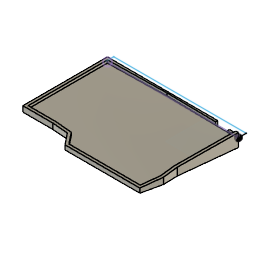
newcase v2 (Autodesk Fusion 360 design; units mm, degrees)
Autodesk Fusion 360 part; units mm, degrees
sketch "board" plane through (0, 0, 0) normal (0, 0, 1) x (1, 0, 0)
  line L0 (-11.43, -11.43) -> (-11.43, 76.4948)
  line L1 (-11.43, 76.4948) -> (53.2209, 77.7986)
  line L2 (53.2209, 77.7986) -> (127.9595, 76.6452)
  line L3 (127.9595, 76.6452) -> (127.335, 12)
  line L4 (127.335, 12) -> (129.2793, -5.0449)
  line L5 (129.2793, -5.0449) -> (126.9476, -25.6233)
  line L6 (126.9476, -25.6233) -> (47.9467, -25.6233)
  line L7 (47.9467, -25.6233) -> (38, -13.05)
  line L8 (38, -13.05) -> (19, -11.43)
  line L9 (19, -11.43) -> (-11.43, -11.43)
  line L10 (130.3366, 12.1561) -> (132.2986, -5.0438)
  line L11 (132.2986, -5.0438) -> (129.6269, -28.6233)
  line L12 (129.6269, -28.6233) -> (46.4947, -28.6233)
  line L13 (46.4947, -28.6233) -> (36.4523, -15.9289)
  line L14 (36.4523, -15.9289) -> (18.8723, -14.43)
  line L15 (18.8723, -14.43) -> (-14.43, -14.43)
  line L16 (-14.43, -14.43) -> (-14.43, 79.4349)
  line L17 (-14.43, 79.4349) -> (53.2138, 80.799)
  line L18 (53.2138, 80.799) -> (130.9882, 79.5988)
  line L19 (130.9882, 79.5988) -> (130.3366, 12.1561)
  line L20 (-35, 100) -> (162.96, 100)
  line L21 (162.96, 100) -> (162.96, -48.8802)
  line L22 (162.96, -48.8802) -> (-35, -48.8802)
  line L23 (-35, -48.8802) -> (-35, 100)
  dimension "d1" = -3
  constraint horizontal L6
  constraint vertical L0
  constraint horizontal L20
  constraint vertical L21
  constraint horizontal L22
  constraint vertical L23
sketch "cutout" plane through (0, 0, 0) normal (0, 0, 1) x (1, 0, 0)
  line L0 (-7.525, -11.025) -> (26.525, -11.025)
  line L1 (-10.525, -8.025) -> (-10.525, 65.025)
  line L2 (-7.525, 68.025) -> (27.475, 68.025)
  line L3 (29.525, -8.025) -> (29.525, -5.025)
  line L4 (29.525, -5.025) -> (43.375, -5.025)
  line L5 (46.475, 74.025) -> (30.475, 74.025)
  line L6 (27.475, 71.025) -> (27.475, 68.025)
  line L7 (67.525, 74.025) -> (67.525, 77.025)
  line L8 (67.525, 77.025) -> (46.475, 77.025)
  line L9 (46.475, 77.025) -> (46.475, 74.025)
  line L10 (86.425, -5.025) -> (87.0325, -5.025)
  line L11 (67.525, 74.025) -> (102.525, 74.025)
  line L12 (105.525, -2.6875) -> (105.525, 0.975)
  line L13 (105.525, 26.025) -> (105.525, 71.025)
  line L14 (105.525, 0.975) -> (107.9545, 0.975)
  line L15 (110.9113, 0.975) -> (121.525, 0.975)
  line L16 (124.525, 3.975) -> (124.525, 20.025)
  line L17 (121.525, 23.025) -> (108.525, 23.025)
  line L18 (49.375, -24.025) -> (86.425, -24.025)
  line L19 (46.375, -8.025) -> (46.375, -21.025)
  line L20 (86.425, -24.025) -> (86.425, -23.1507)
  line L21 (86.425, -11.969) -> (86.425, -5.025)
  line L22 (86.425, -23.1507) -> (103.4355, -24.6389)
  line L23 (106.6855, -21.9118) -> (106.7904, -20.7125)
  line L24 (107.4166, -2.853) -> (105.525, -2.6875)
  line L25 (87.0325, -5.025) -> (86.425, -11.969)
  line L26 (106.7904, -20.7125) -> (122.8174, -22.965)
  line L27 (126.2057, -20.4117) -> (128.4394, -4.5179)
  line L28 (125.8862, -1.1296) -> (110.9113, 0.975)
  line L29 (107.9545, 0.975) -> (107.4166, -2.853)
  arc A0 (26.525, -11.025) -> (29.525, -8.025) centre (26.525, -8.025) ccw
  arc A1 (46.375, -8.025) -> (43.375, -5.025) centre (43.375, -8.025) ccw
  arc A2 (46.375, -21.025) -> (49.375, -24.025) centre (49.375, -21.025) ccw
  arc A3 (103.4355, -24.6389) -> (106.6855, -21.9118) centre (103.6969, -21.6503) ccw
  arc A4 (122.8174, -22.965) -> (126.2057, -20.4117) centre (123.2349, -19.9942) ccw
  arc A5 (128.4394, -4.5179) -> (125.8862, -1.1296) centre (125.4686, -4.1004) ccw
  arc A6 (121.525, 0.975) -> (124.525, 3.975) centre (121.525, 3.975) ccw
  arc A7 (124.525, 20.025) -> (121.525, 23.025) centre (121.525, 20.025) ccw
  arc A8 (105.525, 26.025) -> (108.525, 23.025) centre (108.525, 26.025) ccw
  arc A9 (105.525, 71.025) -> (102.525, 74.025) centre (102.525, 71.025) ccw
  arc A10 (30.475, 74.025) -> (27.475, 71.025) centre (30.475, 71.025) ccw
  arc A11 (-7.525, 68.025) -> (-10.525, 65.025) centre (-7.525, 65.025) ccw
  arc A12 (-10.525, -8.025) -> (-7.525, -11.025) centre (-7.525, -8.025) ccw
  line L30 (-7, -7) -> (7, -7)
  line L31 (7, -7) -> (7, 7)
  line L32 (7, 7) -> (-7, 7)
  line L33 (-7, 7) -> (-7, -7)
  line L34 (-7, 12) -> (7, 12)
  line L35 (7, 12) -> (7, 26)
  line L36 (7, 26) -> (-7, 26)
  line L37 (-7, 26) -> (-7, 12)
  line L38 (-7, 31) -> (7, 31)
  line L39 (7, 31) -> (7, 45)
  line L40 (7, 45) -> (-7, 45)
  line L41 (-7, 45) -> (-7, 31)
  line L42 (-7, 50) -> (7, 50)
  line L43 (7, 50) -> (7, 64)
  line L44 (7, 64) -> (-7, 64)
  line L45 (-7, 64) -> (-7, 50)
  line L46 (12, -7) -> (26, -7)
  line L47 (26, -7) -> (26, 7)
  line L48 (26, 7) -> (12, 7)
  line L49 (12, 7) -> (12, -7)
  line L50 (12, 12) -> (26, 12)
  line L51 (26, 12) -> (26, 26)
  line L52 (26, 26) -> (12, 26)
  line L53 (12, 26) -> (12, 12)
  line L54 (12, 31) -> (26, 31)
  line L55 (26, 31) -> (26, 45)
  line L56 (26, 45) -> (12, 45)
  line L57 (12, 45) -> (12, 31)
  line L58 (12, 50) -> (26, 50)
  line L59 (26, 50) -> (26, 64)
  line L60 (26, 64) -> (12, 64)
  line L61 (12, 64) -> (12, 50)
  line L62 (31, -1) -> (45, -1)
  line L63 (45, -1) -> (45, 13)
  line L64 (45, 13) -> (31, 13)
  line L65 (31, 13) -> (31, -1)
  line L66 (31, 18) -> (45, 18)
  line L67 (45, 18) -> (45, 32)
  line L68 (45, 32) -> (31, 32)
  line L69 (31, 32) -> (31, 18)
  line L70 (31, 37) -> (45, 37)
  line L71 (45, 37) -> (45, 51)
  line L72 (45, 51) -> (31, 51)
  line L73 (31, 51) -> (31, 37)
  line L74 (31, 56) -> (45, 56)
  line L75 (45, 56) -> (45, 70)
  line L76 (45, 70) -> (31, 70)
  line L77 (31, 70) -> (31, 56)
  line L78 (50, 2) -> (64, 2)
  line L79 (64, 2) -> (64, 16)
  line L80 (64, 16) -> (50, 16)
  line L81 (50, 16) -> (50, 2)
  line L82 (50, 21) -> (64, 21)
  line L83 (64, 21) -> (64, 35)
  line L84 (64, 35) -> (50, 35)
  line L85 (50, 35) -> (50, 21)
  line L86 (50, 40) -> (64, 40)
  line L87 (64, 40) -> (64, 54)
  line L88 (64, 54) -> (50, 54)
  line L89 (50, 54) -> (50, 40)
  line L90 (50, 59) -> (64, 59)
  line L91 (64, 59) -> (64, 73)
  line L92 (64, 73) -> (50, 73)
  line L93 (50, 73) -> (50, 59)
  line L94 (69, -1) -> (83, -1)
  line L95 (83, -1) -> (83, 13)
  line L96 (83, 13) -> (69, 13)
  line L97 (69, 13) -> (69, -1)
  line L98 (69, 18) -> (83, 18)
  line L99 (83, 18) -> (83, 32)
  line L100 (83, 32) -> (69, 32)
  line L101 (69, 32) -> (69, 18)
  line L102 (69, 37) -> (83, 37)
  line L103 (83, 37) -> (83, 51)
  line L104 (83, 51) -> (69, 51)
  line L105 (69, 51) -> (69, 37)
  line L106 (69, 56) -> (83, 56)
  line L107 (83, 56) -> (83, 70)
  line L108 (83, 70) -> (69, 70)
  line L109 (69, 70) -> (69, 56)
  line L110 (88, -1) -> (102, -1)
  line L111 (102, -1) -> (102, 13)
  line L112 (102, 13) -> (88, 13)
  line L113 (88, 13) -> (88, -1)
  line L114 (88, 18) -> (102, 18)
  line L115 (102, 18) -> (102, 32)
  line L116 (102, 32) -> (88, 32)
  line L117 (88, 32) -> (88, 18)
  line L118 (88, 37) -> (102, 37)
  line L119 (102, 37) -> (102, 51)
  line L120 (102, 51) -> (88, 51)
  line L121 (88, 51) -> (88, 37)
  line L122 (88, 56) -> (102, 56)
  line L123 (102, 56) -> (102, 70)
  line L124 (102, 70) -> (88, 70)
  line L125 (88, 70) -> (88, 56)
  line L126 (107, 5) -> (121, 5)
  line L127 (121, 5) -> (121, 19)
  line L128 (121, 19) -> (107, 19)
  line L129 (107, 19) -> (107, 5)
  line L130 (49.9, -20) -> (63.9, -20)
  line L131 (63.9, -20) -> (63.9, -6)
  line L132 (63.9, -6) -> (49.9, -6)
  line L133 (49.9, -6) -> (49.9, -20)
  line L134 (68.9, -20) -> (82.9, -20)
  line L135 (82.9, -20) -> (82.9, -6)
  line L136 (82.9, -6) -> (68.9, -6)
  line L137 (68.9, -6) -> (68.9, -20)
  line L138 (89.3165, -19.3633) -> (103.2633, -20.5835)
  line L139 (103.2633, -20.5835) -> (104.4835, -6.6367)
  line L140 (104.4835, -6.6367) -> (90.5367, -5.4165)
  line L141 (90.5367, -5.4165) -> (89.3165, -19.3633)
  line L142 (108.9939, -16.9577) -> (122.8577, -18.9061)
  line L143 (122.8577, -18.9061) -> (124.8061, -5.0423)
  line L144 (124.8061, -5.0423) -> (110.9423, -3.0939)
  line L145 (110.9423, -3.0939) -> (108.9939, -16.9577)
extrude "Extrude1" add sketch "board" along normal blind 5 contours L10 L11 L12 L13 L14 L15 L16 L17 L18 L19
sketch "Sketch3" plane through (0, 0, 5) normal (0, 0, 1) x (-1, 0, 0)
  line L0 (-38, 13.05) -> (-19, 11.43)
  line L1 (-19, 11.43) -> (11.43, 11.43)
  line L2 (11.43, 11.43) -> (11.43, -76.4948)
  line L3 (11.43, -76.4948) -> (-53.2209, -77.7986)
  line L4 (-53.2209, -77.7986) -> (-127.9595, -76.6452)
  line L5 (-127.9595, -76.6452) -> (-127.335, -12)
  line L6 (-127.335, -12) -> (-129.2793, 5.0449)
  line L7 (-129.2793, 5.0449) -> (-126.9476, 25.6233)
  line L8 (-126.9476, 25.6233) -> (-47.9467, 25.6233)
  line L9 (-47.9467, 25.6233) -> (-38, 13.05)
  line L10 (-130.9882, -79.5988) -> (-53.2138, -80.799)
  line L11 (-53.2138, -80.799) -> (14.43, -79.4349)
  line L12 (14.43, -79.4349) -> (14.43, 14.43)
  line L13 (14.43, 14.43) -> (-18.8723, 14.43)
  line L14 (-18.8723, 14.43) -> (-36.4523, 15.9289)
  line L15 (-36.4523, 15.9289) -> (-46.4947, 28.6233)
  line L16 (-46.4947, 28.6233) -> (-129.6269, 28.6233)
  line L17 (-129.6269, 28.6233) -> (-132.2986, 5.0438)
  line L18 (-132.2986, 5.0438) -> (-130.3366, -12.1561)
  line L19 (-130.3366, -12.1561) -> (-130.9882, -79.5988)
  line L20 (-107.9906, -79.9537) -> (-107.9443, -76.9541)
  line L21 (-127.9882, -79.6451) -> (-127.9419, -76.6455)
  dimension "d21" = 20
  dimension "d22" = 3
  constraint coincident L10 L20.start
  constraint coincident L4 L20.end
  constraint perpendicular L4 L20
  constraint coincident L10 L21.start
  constraint coincident L4 L21.end
  constraint perpendicular L4 L21
  measures "d21" distance of L20 L21
  measures "d22" horizontal distance of L10.start L21.start
extrude "Extrude2" cut sketch "Sketch3" against normal blind 2 contours L4 L10 L20 L21
extrude "Extrude3" add sketch "board" 1 faces at (-13.43, 17.8583, 0) along normal blind 2 contours L0 L1 L2 L3 L4 L5 L6 L7 L8 L9
sketch "Sketch4" plane through (-14.43, 0, 0) normal (-1, 0, 0) x (0, -1, 0)
  line L0 (14.43, 0) -> (14.43, 5)
  line L1 (14.43, 5) -> (-79.4349, 5)
  line L2 (-79.4349, 5) -> (-79.4349, 0)
  line L3 (-79.4349, 0) -> (14.43, 0)
  line L4 (28.6233, 0) -> (28.6233, 5)
  line L5 (-79.4349, 0) -> (-79.4349, -9.4249)
  line L6 (-79.4349, -9.4249) -> (28.6233, 0)
  line L7 (-79.4349, 0) -> (-34.4349, 0) construction
  line L8 (-34.4349, 0) -> (-34.4349, -5.5)
  line L9 (28.6233, 0) -> (15.9289, 0)
  line L10 (15.9289, 0) -> (14.43, 0)
  dimension "d8" = 45
  dimension "d9" = 5.5
  constraint coincident L2.end L3.start
  constraint perpendicular L3 L5
  constraint coincident L4.start L6.end
  constraint perpendicular L5 L7
  constraint perpendicular L7 L8
  constraint coincident L6 L8.end
  measures "d8" distance of L2.end L7.end
  measures "d9" distance of L7.end L8.end
extrude "Extrude4" add sketch "Sketch4" against normal blind 150 contours L3 L6 L8 L9 L10 | L3 L5 L6 L8
extrude "Extrude5" cut sketch "board" against normal blind 15 contours L20 L21 L22 L23
sketch "Sketch5" plane through (0, 79.4349, 0) normal (0, 1, 0) x (-1, 0, 0)
  line L0 (-130.9866, 0) -> (-130.9866, -9.4249)
  line L1 (-130.9866, -9.4249) -> (14.43, -9.4249)
  line L2 (14.43, -9.4249) -> (14.43, 0)
  line L3 (14.43, 0) -> (-130.9866, 0)
  line L4 (-120.9866, 0) -> (-93.9866, 0)
  line L5 (-93.9866, 0) -> (-93.9866, -5)
  line L6 (-93.9866, -5) -> (-120.9866, -5)
  line L7 (-120.9866, -5) -> (-120.9866, 0)
  line L8 (35, 0) -> (-162.96, 0)
  dimension "d14" = 27
  dimension "d15" = 10
  dimension "d16" = 5
  constraint horizontal L4
  constraint vertical L5
  constraint horizontal L6
  constraint vertical L7
  constraint coincident L3 L4.start
  measures "d14" distance of L4.start L4.end
  measures "d15" distance of L0 L7
  measures "d16" distance of L6 L8
extrude "Extrude6" cut sketch "Sketch5" against normal blind 44 contours L3 L4 L5 L6 L7 L8
sketch "Sketch7" plane through (1.2593, 81.6008, 0) normal (0.01543, 0.999881, 0) x (-0.999881, 0.01543, 0)
  line L0 (-51.9607, 0) -> (-51.9607, 5)
  line L1 (-51.9607, 5) -> (-106.744, 5)
  line L2 (-106.744, 5) -> (-106.744, 3)
  line L3 (-106.744, 3) -> (-126.744, 3)
  line L4 (-126.744, 3) -> (-126.744, 5)
  line L5 (-126.744, 5) -> (-129.7444, 5)
  line L6 (-129.7444, 5) -> (-129.7444, 0)
  line L7 (-129.7444, 0) -> (-51.9607, 0)
  line L8 (-119.7465, -5) -> (-119.7465, 0)
  line L9 (-119.7465, 0) -> (-119.7465, 3)
  line L10 (-106.744, 3) -> (-106.744, 0)
  constraint coincident L8.end L9.start
  constraint coincident L3 L9.end
  constraint perpendicular L3 L9
  constraint coincident L2.end L3.start
  constraint coincident L7 L10.end
  constraint perpendicular L7 L10
extrude "Extrude7" cut sketch "Sketch7" against normal blind 3 contours L3 L7 L9 L10
sketch "Sketch8" plane through (0, 0, 0) normal (0, 0, -1) x (1, 0, 0)
  line L0 (107.9906, -79.9537) -> (107.9443, -76.9541)
  line L1 (107.9443, -76.9541) -> (120.9452, -76.7534)
  line L2 (120.9452, -76.7534) -> (120.9866, -79.4349)
  line L3 (120.9866, -79.4349) -> (120.9866, -35.4349)
  line L4 (120.9866, -35.4349) -> (93.9866, -35.4349)
  line L5 (93.9866, -35.4349) -> (93.9866, -79.4349)
  line L6 (93.9866, -79.4349) -> (-14.43, -79.4349)
  line L7 (-14.43, -79.4349) -> (53.2138, -80.799)
  line L8 (53.2138, -80.799) -> (107.9906, -79.9537)
  line L9 (-14.43, -79.4349) -> (130.9866, -79.4349)
  line L10 (130.9866, -79.4349) -> (-16, -79.4349)
  line L11 (-16, -79.4349) -> (-16, -88)
  line L12 (-16, -88) -> (130.9866, -88)
  line L13 (130.9866, -88) -> (130.9866, -79.4349)
  constraint horizontal L10
  constraint vertical L11
  constraint horizontal L12
  constraint vertical L13
  constraint coincident L9.end L10.start
extrude "Extrude8" cut sketch "Sketch8" against normal blind 7 contours L0 L7 L8 L9 L10 L11 L12 L13
extrude "Extrude9" cut sketch "Sketch8" against normal blind 10 contours L0 L6 L7 L8 L9 L10 | L0 L7 L8 L9 L10 L11 L12 L13
